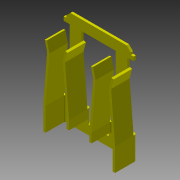
# Autodesk Inventor part: SNT-100_pins
Saved by Autodesk Inventor 2014 SP2 (Build 180246200, 246)
## iProperties
Created: 2019-03-13
Part Number: SNT-100_pins
Material: Generic
Catalog Web Link: www.cadenas.de
Description: SNT Pins-SNT Series - (2,54 mm) .100" Shunt
Vendor: SAMTEC
Document SubType Name: Modeling
Designer: psadmin
Manufacturer: SAMTEC
Mass: 0.00345016 g
Surface Area: 0.62771 cm^2
Volume: 0.00345016 cm^3
Density: 1 g/cm^3
Appearance: PSOLRGB-255-255-0
Category: PARTsolutions
Company: SAMTEC
Title: SNT-100_pins
Author: Cadenas PARTsolutions
Comments: SNT Series - (2,54 mm) .100" Shunt
PSOL_IDENT_0: {$CADENAS_DATA\23d-libs\samtec\modelling\snt\parts\snt_pins.prj},166 {VTYP=3D},{NB=SNT-100_pins},{LI
PSOL_IDENT_1: NA=SNT-100_pins},{NN=SNT Pins},{DATE=22.01.2016 08:16:46},{GEOMDATE=20.01.2016 06:57:00},{VERSION=},
PSOL_IDENT_2: {LINEID=10},{WBVAR=},{WBNUMERIC=}  {NB=SNT-100_pins},{LINA=SNT-100_pins},{KT=DUMMY},{PN=SNT-100},{SE
PSOL_IDENT_3: RIES=SNT},{A=0.240},{W=0.100},{L=0.200},{PINW=0.040}
NN: SNT Pins
NT: SNT Series - (2,54 mm) .100" Shunt
NB: SNT-100_pins
NBSYN: $PN._pins
LINA: SNT-100_pins
PN: SNT-100
SERIES: SNT
A: 0.24
W: 0.1
L: 0.2
PINW: 0.04
SUPPLIER: SAMTEC
ARTICLENO: SNT-100_pins
BOMINFO: SNT-100_pins
CREATOR: CADENAS GmbH
Autodesk Inventor part; units mm, degrees
ref_plane "YZ Plane" through (0, 0, 0) normal (1, 0, 0) x (0, 1, 0)
ref_plane "XZ Plane" through (0, 0, 0) normal (0, 1, 0) x (-1, 0, 0)
ref_plane "XY Plane" through (0, 0, 0) normal (0, 0, 1) x (1, 0, 0)
sketch "Sketch__1" plane through (0, 0, -0.508) normal (0, 0, 1) x (1, 0, 0)
  line L0 (-1.9125, 5.4482) -> (-1.9125, 5.2322)
  line L1 (-1.9125, 5.2322) -> (-1.5875, 5.2322)
  line L2 (-1.5875, 5.2322) -> (-1.5875, 0.4572)
  line L3 (-1.5875, 0.4572) -> (1.5875, 0.4572)
  line L4 (1.5875, 0.4572) -> (1.5875, 5.2322)
  line L5 (1.5875, 5.2322) -> (1.9295, 5.2322)
  line L6 (1.9295, 5.2322) -> (1.9295, 5.4482)
  line L7 (1.9295, 5.4482) -> (1.7775, 5.4482)
  line L8 (1.7775, 5.4482) -> (1.7775, 5.5632)
  line L9 (1.7775, 5.5632) -> (1.5485, 5.7912)
  line L10 (1.5485, 5.7912) -> (-1.5495, 5.7912)
  line L11 (-1.5495, 5.7912) -> (-1.7785, 5.5632)
  line L12 (-1.7785, 5.5632) -> (-1.7785, 5.4482)
  line L13 (-1.7785, 5.4482) -> (-1.9125, 5.4482)
  line L14 (-0.9525, 0.9652) -> (0.9525, 0.9652)
  line L15 (0.9525, 0.9652) -> (0.9525, 5.2322)
  line L16 (0.9525, 5.2322) -> (-0.9525, 5.2322)
  line L17 (-0.9525, 5.2322) -> (-0.9525, 0.9652)
  constraints: 36 end point
extrude "Extrusion1" add sketch "Sketch__1" against normal blind 0.127
sketch "Sketch_1" plane through (0, 0.4572, 0) normal (0, 1, 0) x (1, 0, 0)
  line L0 (0.5588, 0.508) -> (0.5588, 0.4572)
  line L1 (0.5588, 0.4572) -> (0.6858, 0.4572)
  arc A0 (0.7366, 0.508) -> (0.6858, 0.4572) centre (0.7366, 0.4572) ccw
  line L2 (0.7366, 0.508) -> (1.8034, 0.508)
  arc A1 (1.8542, 0.4572) -> (1.8034, 0.508) centre (1.8034, 0.4572) ccw
  line L3 (1.8542, 0.4572) -> (1.8542, -0.5588)
  line L4 (1.8542, -0.5588) -> (1.9812, -0.5588)
  line L5 (1.9812, -0.5588) -> (1.9812, 0.508)
  arc A2 (1.9812, 0.508) -> (1.8542, 0.635) centre (1.8542, 0.508) ccw
  line L6 (1.8542, 0.635) -> (0.6858, 0.635)
  arc A3 (0.6858, 0.635) -> (0.5588, 0.508) centre (0.6858, 0.508) ccw
  constraints: 14 end point, 8 point on circle, 4 centre point
extrude "Extrusion2" add sketch "Sketch_1" along normal blind 1.27
sketch "Sketch_2" plane through (0, 0.4572, 0) normal (0, 1, 0) x (1, 0, 0)
  line L0 (-1.9812, 0.508) -> (-1.9812, -0.5588)
  line L1 (-1.9812, -0.5588) -> (-1.8542, -0.5588)
  line L2 (-1.8542, -0.5588) -> (-1.8542, 0.4572)
  arc A0 (-1.8034, 0.508) -> (-1.8542, 0.4572) centre (-1.8034, 0.4572) ccw
  line L3 (-1.8034, 0.508) -> (-0.7366, 0.508)
  arc A1 (-0.6858, 0.4572) -> (-0.7366, 0.508) centre (-0.7366, 0.4572) ccw
  line L4 (-0.6858, 0.4572) -> (-0.5588, 0.4572)
  line L5 (-0.5588, 0.4572) -> (-0.5588, 0.508)
  arc A2 (-0.5588, 0.508) -> (-0.6858, 0.635) centre (-0.6858, 0.508) ccw
  line L6 (-0.6858, 0.635) -> (-1.8542, 0.635)
  arc A3 (-1.8542, 0.635) -> (-1.9812, 0.508) centre (-1.8542, 0.508) ccw
  constraints: 14 end point, 8 point on circle, 4 centre point
extrude "Extrusion3" add sketch "Sketch_2" along normal blind 1.27
sketch "Sketch_3" plane through (0, 0.4572, 0) normal (0, 1, 0) x (1, 0, 0)
  line L0 (-0.8128, 0.508) -> (-0.8128, -0.508)
  line L1 (-0.8128, -0.508) -> (0.8128, -0.508)
  line L2 (0.8128, -0.508) -> (0.8128, 0.508)
  line L3 (0.8128, 0.508) -> (-0.8128, 0.508)
  constraints: 8 end point
extrude "Extrusion4" cut sketch "Sketch_3" along normal blind 0.762
sketch "Sketch_4" plane through (0, 0, -0.4572) normal (0, 0, 1) x (1, 0, 0)
  line L0 (-1.9812, 1.7272) -> (-1.9812, 1.2192)
  line L1 (-1.9812, 1.2192) -> (-0.5588, 1.2192)
  line L2 (-0.5588, 1.2192) -> (-0.5588, 1.7272)
  line L3 (-0.5588, 1.7272) -> (-0.7741, 4.3308)
  arc A0 (-0.7707, 4.3772) -> (-0.7741, 4.3308) centre (-0.635, 4.3437) ccw
  line L4 (-0.7707, 4.3772) -> (-0.643, 4.8715)
  line L5 (-0.643, 4.8715) -> (-0.762, 4.9022)
  line L6 (-0.762, 4.9022) -> (-0.8973, 4.3783)
  arc A1 (-0.8973, 4.3783) -> (-0.9012, 4.3319) centre (-0.762, 4.3434) ccw
  line L7 (-0.9012, 4.3319) -> (-0.6858, 1.7272)
  line L8 (-0.6858, 1.7272) -> (-0.6858, 1.2954)
  line L9 (-0.6858, 1.2954) -> (-1.8542, 1.2954)
  line L10 (-1.8542, 1.2954) -> (-1.8542, 1.7272)
  line L11 (-1.8542, 1.7272) -> (-1.6388, 4.3319)
  arc A2 (-1.6388, 4.3319) -> (-1.6427, 4.3783) centre (-1.778, 4.3434) ccw
  line L12 (-1.6427, 4.3783) -> (-1.778, 4.9022)
  line L13 (-1.778, 4.9022) -> (-1.897, 4.8715)
  line L14 (-1.897, 4.8715) -> (-1.7693, 4.3772)
  arc A3 (-1.7659, 4.3308) -> (-1.7693, 4.3772) centre (-1.905, 4.3437) ccw
  line L15 (-1.7659, 4.3308) -> (-1.9812, 1.7272)
  constraints: 32 end point, 8 point on circle, 4 centre point
extrude "Extrusion5" add sketch "Sketch_4" along normal blind 1.016
sketch "Sketch_5" plane through (0, 0, -0.4572) normal (0, 0, 1) x (1, 0, 0)
  line L0 (0.5588, 1.7272) -> (0.5588, 1.2192)
  line L1 (0.5588, 1.2192) -> (1.9812, 1.2192)
  line L2 (1.9812, 1.2192) -> (1.9812, 1.7272)
  line L3 (1.9812, 1.7272) -> (1.7659, 4.3308)
  arc A0 (1.7693, 4.3772) -> (1.7659, 4.3308) centre (1.905, 4.3437) ccw
  line L4 (1.7693, 4.3772) -> (1.897, 4.8715)
  line L5 (1.897, 4.8715) -> (1.778, 4.9022)
  line L6 (1.778, 4.9022) -> (1.6427, 4.3783)
  arc A1 (1.6427, 4.3783) -> (1.6388, 4.3319) centre (1.778, 4.3434) ccw
  line L7 (1.6388, 4.3319) -> (1.8542, 1.7272)
  line L8 (1.8542, 1.7272) -> (1.8542, 1.2954)
  line L9 (1.8542, 1.2954) -> (0.6858, 1.2954)
  line L10 (0.6858, 1.2954) -> (0.6858, 1.7272)
  line L11 (0.6858, 1.7272) -> (0.9012, 4.3319)
  arc A2 (0.9012, 4.3319) -> (0.8973, 4.3783) centre (0.762, 4.3434) ccw
  line L12 (0.8973, 4.3783) -> (0.762, 4.9022)
  line L13 (0.762, 4.9022) -> (0.643, 4.8715)
  line L14 (0.643, 4.8715) -> (0.7707, 4.3772)
  arc A3 (0.7741, 4.3308) -> (0.7707, 4.3772) centre (0.635, 4.3437) ccw
  line L15 (0.7741, 4.3308) -> (0.5588, 1.7272)
  constraints: 32 end point, 8 point on circle, 4 centre point
extrude "Extrusion6" add sketch "Sketch_5" along normal blind 1.016
sketch "Sketch_6" plane through (0, 0, -0.4572) normal (0, 0, 1) x (1, 0, 0)
  line L0 (-1.8542, 1.397) -> (-1.8542, 0)
  line L1 (-1.8542, 0) -> (1.8542, 0)
  line L2 (1.8542, 0) -> (1.8542, 1.397)
  line L3 (1.8542, 1.397) -> (0.6858, 1.397)
  line L4 (0.6858, 1.397) -> (0.6858, 0.0762)
  line L5 (0.6858, 0.0762) -> (-0.6858, 0.0762)
  line L6 (-0.6858, 0.0762) -> (-0.6858, 1.397)
  line L7 (-0.6858, 1.397) -> (-1.8542, 1.397)
  constraints: 16 end point
extrude "Extrusion7" cut sketch "Sketch_6" along normal blind 1.27
ref_plane "pins_to_body_XY" through (0, 0, -0.0381) normal (0, 1, 0) x (1, 0, 0)
ref_plane "pins_to_body_YZ" through (0, 0, -0.0381) normal (1, 0, 0) x (0, 0, -1)
ref_plane "pins_to_body_ZX" through (0, 0, -0.0381) normal (0, 0, -1) x (0, 1, 0)
body "Solid1"
